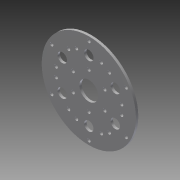
# Autodesk Inventor part: Plate (Front)
Saved by Autodesk Inventor 2014 (Build 180170000, 170)
## iProperties
Created: 2014-01-12
Part Number: Plate (Front)
Material: Steel
Document SubType Name: Sheet Metal
Designer: Andrew Toennies
Mass: 273.498 g
Surface Area: 253.67 cm^2
Volume: 34.8405 cm^3
Density: 7.85 g/cm^3
Sheet Metal Rule: Default
Appearance: Steel
Author: Andrew Toennies
Autodesk Inventor part; units mm, degrees
ref_plane "YZ Plane" through (0, 0, 0) normal (1, 0, 0) x (0, 1, 0)
ref_plane "XZ Plane" through (0, 0, 0) normal (0, 1, 0) x (-1, 0, 0)
ref_plane "XY Plane" through (0, 0, 0) normal (0, 0, 1) x (1, 0, 0)
sketch "Sketch1" plane through (0, 0, 0) normal (0, 0, 1) x (1, 0, 0)
  circle A0 centre (0, 0) radius 63.5
  circle A1 centre (0, 0) radius 12.7
  circle A2 centre (0, 41.275) radius 6.35
  line L0 (0, 0) -> (0, 41.275) construction
  line L1 (0, 41.275) -> (0, 57.9438) construction
  line L2 (-16.6688, 41.275) -> (16.6688, 41.275) construction
  circle A3 centre (-35.7452, 20.6375) radius 6.35
  circle A4 centre (-35.7452, -20.6375) radius 6.35
  circle A5 centre (0, -41.275) radius 6.35
  circle A6 centre (35.7452, -20.6375) radius 6.35
  circle A7 centre (35.7452, 20.6375) radius 6.35
  dimension "d0" = 127
  dimension "d1" = 25.4
  dimension "d2" = 12.7
  dimension "d3" = 41.275
  dimension "d22" = 360
  constraints: 8 centre point, 6 end point, 3 coincident, 2 vertical, 1 midpoint, 1 perpendicular, 13 other
  measures "d0" diameter of A0
  measures "d1" diameter of A1
  measures "d2" diameter of A2
  measures "d3" distance of L0.start L0.end
extrude "Plate2" add sketch "Sketch1" along normal blind 3.175
equation "\"BendRadius\" = Thickness"
equation "\"BendReliefWidth\" = Thickness"
equation "\"BendReliefDepth\" = 0.5 * Thickness"
equation "\"CornerReliefSize\" = 4 * Thickness"
equation "\"MinimumRemnant\" = 2 * Thickness"
equation "\"TransitionRadius\" = BendRadius"
equation "\"JacobiRadiusSize\" = BendRadius"
equation "\"GapSize\" = Thickness"
equation "\"d8\" = BendRadius"
equation "\"d19\" = BendRadius"
equation "\"Thickness\" = 3.175"
body "Solid2"
